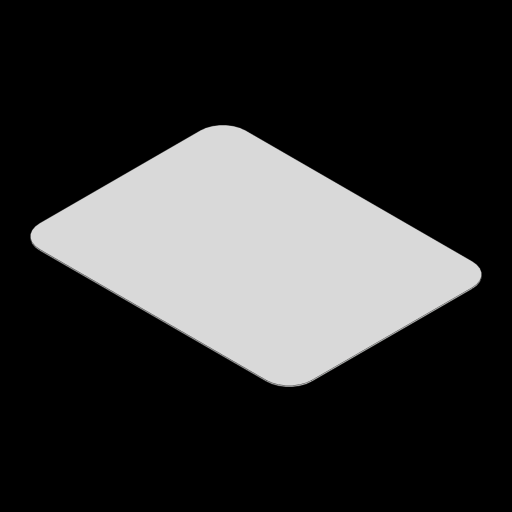
# Autodesk Inventor part: 230_Diffuser
Saved by Autodesk Inventor 2024 (Build 280153000, 153)
## iProperties
Created: 2023-07-20
Part Number: 230_Diffuser
Material: Generisch
Document SubType Name: Modeling
Designer: Philipp
Density: 1 g/cm^3
Appearance: Vorgabe
Author: Philipp
Autodesk Inventor part; units mm, degrees
ref_plane "YZ Plane" through (0, 0, 0) normal (1, 0, 0) x (0, 1, 0)
ref_plane "XZ Plane" through (0, 0, 0) normal (0, 1, 0) x (-1, 0, 0)
ref_plane "XY Plane" through (0, 0, 0) normal (0, 0, 1) x (1, 0, 0)
sketch "Skizze1" plane through (0, 0, 0) normal (0, 0, 1) x (1, 0, 0)
  line L0 (-72, 54.5) -> (72, 54.5)
  line L1 (72, 54.5) -> (72, -54.5)
  line L2 (72, -54.5) -> (-72, -54.5)
  line L3 (-72, -54.5) -> (-72, 54.5)
  line L4 (-72, 54.5) -> (72, -54.5) construction
  line L5 (72, 54.5) -> (-72, -54.5) construction
  point P0 (0, 0)
  dimension "d0" = 144
  dimension "d1" = 109
  constraints: 12 end point, 2 midpoint, 2 parallel, 1 horizontal, 1 perpendicular
  measures "d0" distance of L1.end L2.end
  measures "d1" distance of L0.end L1.end
extrude "Extrusion1" add sketch "Skizze1" along normal blind 0.6
fillet "Rundung1" radius 12 4 edges at (72, 54.5, 0.3) (72, -54.5, 0.3) (-72, -54.5, 0.3) (-72, 54.5, 0.3)
